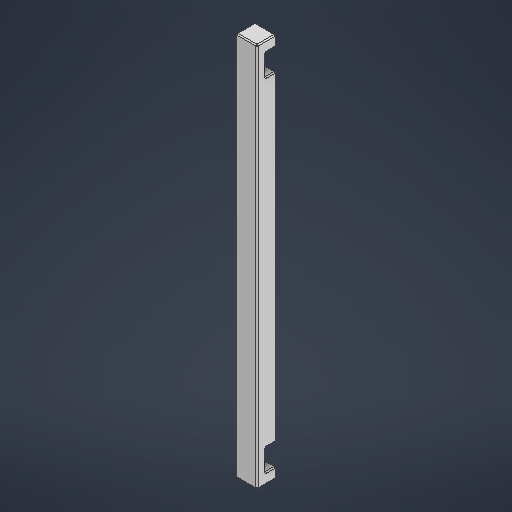
# Autodesk Inventor part: LegsStabilizer
Saved by Autodesk Inventor 2026.3 (Build 303398000, 398)
## iProperties
Created: 2026-05-02
Part Number: LegsStabilizer
Material: Generic
Document SubType Name: Modeling
Designer: frede
Density: 1 g/cm^3
Appearance: Default
Author: frede
Autodesk Inventor part; units mm, degrees
ref_plane "YZ Plane" through (0, 0, 0) normal (1, 0, 0) x (0, 1, 0)
ref_plane "XZ Plane" through (0, 0, 0) normal (0, 1, 0) x (-1, 0, 0)
ref_plane "XY Plane" through (0, 0, 0) normal (0, 0, 1) x (1, 0, 0)
sketch "Sketch1" plane through (0, 0, 0) normal (1, 0, 0) x (0, 1, 0)
  line L0 (0, 0) -> (181, 0)
  line L1 (181, 0) -> (181, -9)
  line L2 (0, -9) -> (0, 0)
  line L3 (15.1, -9) -> (15.1, -4)
  line L4 (15.1, -4) -> (5, -4)
  line L5 (5, -4) -> (5, -9)
  line L6 (165.9, -9) -> (165.9, -4)
  line L7 (165.9, -4) -> (176, -4)
  line L8 (176, -4) -> (176, -9)
  line L9 (5, -9) -> (0, -9)
  line L10 (181, -9) -> (176, -9)
  line L11 (165.9, -9) -> (15.1, -9)
  dimension "d0" = 181
  dimension "d1" = 10.1
  dimension "d3" = 10.1
  dimension "d5" = 5
  dimension "d7" = 5
  dimension "d8" = 5
  dimension "d11" = 9
  dimension "d12" = 171
  dimension "d17" = 9
  dimension "d18" = 9
  constraints: 24 end point, 6 parallel, 1 horizontal, 1 perpendicular
  measures "d0" distance of L1.end L2.start
  measures "d1" distance of L4.end L3.end
  measures "d3" distance of L6.end L7.end
  measures "d5" distance between parallel lines of L8 L1
  measures "d7" distance between parallel lines of L11 L7
  measures "d8" distance between parallel lines of L11 L4
  measures "d11" distance between parallel lines of L0 L11
  measures "d12" distance between parallel lines of L8 L5
  measures "d17" distance between parallel lines of L0 L10
  measures "d18" distance between parallel lines of L0 L9
extrude "Extrusion1" add sketch "Sketch1" along normal blind 9.9
fillet "Fillet1" radius 0.5 4 edges at (4.95, 176, -4) (4.95, 165.9, -4) (4.95, 15.1, -4) (4.95, 5, -4)
chamfer "Chamfer1" distance 0.5 angle 45 40 edges at (9.9, 90.5, 0) (9.9, 90.5, -9) (9.9, 15.1, -6.75) (9.9, 14.9536, -4.1464) (9.9, 10.05, -4) (9.9, 5.1464, -4.1464) (9.9, 5, -6.75) (9.9, 0, -4.5) (9.9, 2.5, -9) (4.95, 0, -9) (0, 0, -4.5) (4.95, 0, 0) (0, 90.5, 0) (9.9, 176, -6.75) (9.9, 175.8536, -4.1464) (9.9, 170.95, -4) (9.9, 166.0464, -4.1464) (9.9, 165.9, -6.75) (9.9, 178.5, -9) (9.9, 181, -4.5) (0, 181, -4.5) (0, 178.5, -9) (4.95, 176, -9) (4.95, 181, -9) (4.95, 181, 0) (4.95, 15.1, -9) (4.95, 165.9, -9) (0, 170.95, -4) (0, 175.8536, -4.1464) (0, 176, -6.75) (0, 166.0464, -4.1464) (0, 165.9, -6.75) (0, 90.5, -9) (0, 15.1, -6.75) (0, 14.9536, -4.1464) (0, 10.05, -4) (0, 5.1464, -4.1464) (0, 5, -6.75) (0, 2.5, -9) (4.95, 5, -9)
equation "\"d5\" = -0.5 * d12 + 0.5 * d0"
equation "\"d17\" = d11"
equation "\"d18\" = d17"
body "Solid1"
